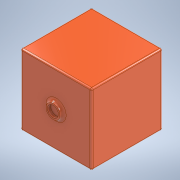
# Autodesk Inventor part: Kamera
Saved by Autodesk Inventor 2020 (Build 240168000, 168)
## iProperties
Created: 2021-10-14
Part Number: Kamera
Material: Ogólny
Document SubType Name: Modeling
Designer: Komputer
Density: 1 g/cm^3
Appearance: Gładki — jasnopomarańczowy
Author: Komputer
Autodesk Inventor part; units mm, degrees
ref_plane "YZ Plane" through (0, 0, 0) normal (1, 0, 0) x (0, 1, 0)
ref_plane "XZ Plane" through (0, 0, 0) normal (0, 1, 0) x (-1, 0, 0)
ref_plane "XY Plane" through (0, 0, 0) normal (0, 0, 1) x (1, 0, 0)
sketch "Szkic1" plane through (0, 0, 0) normal (0, 0, 1) x (1, 0, 0)
  line L0 (11.5, -11.5) -> (-11.5, -11.5)
  line L1 (-11.5, -11.5) -> (-11.5, 11.5)
  line L2 (-11.5, 11.5) -> (11.5, 11.5)
  line L3 (11.5, 11.5) -> (11.5, -11.5)
  line L4 (11.5, -11.5) -> (-11.5, 11.5) construction
  line L5 (-11.5, -11.5) -> (11.5, 11.5) construction
  point P0 (0, 0)
  dimension "d0" = 23
  dimension "d1" = 23
  constraints: 12 end point, 2 midpoint, 2 parallel, 1 horizontal, 1 perpendicular
  measures "d0" distance of L1.end L2.end
  measures "d1" distance of L0.end L1.end
extrude "Wyciągnięcie proste1" add sketch "Szkic1" along normal blind 23
fillet "Zaokrąglenie1" radius 0.5 12 edges at (0, 11.5, 23) (11.5, 11.5, 11.5) (11.5, 0, 23) (11.5, 0, 0) (11.5, -11.5, 11.5) (0, -11.5, 23) (0, -11.5, 0) (-11.5, -11.5, 11.5) (0, 11.5, 0) (-11.5, 11.5, 11.5) (-11.5, 0, 0) (-11.5, 0, 23)
sketch "Szkic2" plane through (0, 0, 23) normal (0, 0, 1) x (1, 0, 0)
  circle A0 centre (0, 0) radius 1.75
  circle A1 centre (0, 0) radius 2.25
  dimension "d5" = 3.5
  dimension "d6" = 4.5
  constraints: 2 centre point, 2 coincident
  measures "d5" diameter of A0
  measures "d6" diameter of A1
extrude "Wyciągnięcie proste2" add sketch "Szkic2" along normal blind 1
fillet "Zaokrąglenie2" radius 1 1 edges at (-2.25, 0, 23)
